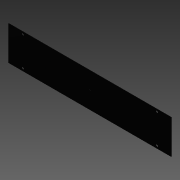
# Autodesk Inventor part: Sheild Flat
Saved by Autodesk Inventor 2014 SP1 (Build 180222100, 222)
## iProperties
Created: 2014-01-13
Part Number: Sheild Flat
Material: Aluminum 6061
Document SubType Name: Sheet Metal
Designer: Rauhul Varma
Mass: 21.0227 g
Surface Area: 199.954 cm^2
Volume: 7.75744 cm^3
Density: 2.71 g/cm^3
Sheet Metal Rule: Default
Appearance: Anodized - Black
Author: Rauhul Varma
Autodesk Inventor part; units mm, degrees
ref_plane "YZ Plane" through (0, 0, 0) normal (1, 0, 0) x (0, 1, 0)
ref_plane "XZ Plane" through (0, 0, 0) normal (0, 1, 0) x (-1, 0, 0)
ref_plane "XY Plane" through (0, 0, 0) normal (0, 0, 1) x (1, 0, 0)
sketch "Sketch1" plane through (0, 0, 0) normal (0, 0, 1) x (1, 0, 0)
  line L0 (0, 0) -> (216.6575, 0)
  line L1 (216.6575, 0) -> (216.6575, 45.2438)
  line L2 (216.6575, 45.2438) -> (0, 45.2437)
  line L3 (0, 45.2437) -> (0, 0)
  dimension "d0" = 216.6575
  dimension "d1" = 45.2437
  measures "d0" distance of L1.end L2.end
  measures "d1" distance of L2.end L0.start
extrude "Plate1" add sketch "Sketch1" along normal blind 0.7937
sketch "Sketch2" plane through (0, 0, 0) normal (0, 0, -1) x (-1, 0, 0)
  line L0 (0, 0) -> (-216.6575, 0) projected
  line L1 (0, 45.2437) -> (0, 0) projected
  line L2 (-216.6575, 45.2438) -> (0, 45.2437) projected
  line L3 (-216.6575, 0) -> (-216.6575, 45.2438) projected
  line L4 (-197.6075, 45.2438) -> (-197.6075, 0) construction
  line L5 (-216.6575, 3.175) -> (0, 3.175) construction
  line L6 (-19.05, 0) -> (-19.05, 45.2437) construction
  line L7 (0, 42.0687) -> (-216.6575, 42.0688) construction
  point P0 (-197.6075, 42.0688)
  point P1 (-197.6075, 3.175)
  point P2 (-19.05, 3.175)
  point P3 (-19.05, 42.0687)
  point P4 (-108.3288, 22.6219)
  dimension "d3" = 3.175
  dimension "d4" = 3.175
  dimension "d5" = 19.05
  dimension "d6" = 19.05
  dimension "d7" = 22.6219
  dimension "d8" = 108.3288
  dimension "d9" = 45.2437
  dimension "d10" = 216.6575
  constraints: 16 point on line, 8 end point, 3 perpendicular, 1 horizontal
  measures "d3" distance between parallel lines of L2 L7
  measures "d4" distance between parallel lines of L0 L5
  measures "d5" distance between parallel lines of L3 L4
  measures "d6" distance between parallel lines of L1 L6
  measures "d7" distance from line of L2 point (-108.329, 22.622)
  measures "d8" distance from line of L1 point (-108.329, 22.622)
  measures "d9" distance of L1.start L0.start
  measures "d10" distance of L2.start L1.start
hole "Hole1" at (197.6075, 42.0688, 0) at (197.6075, 3.175, 0) at (19.05, 3.175, 0) at (19.05, 42.0687, 0) direction (0, 0, 1) diameter 2.9464 end through all clearance for "Flat Head Machine Screw (82)" size "#4" standard "Ansi Unified Screw Threads"
hole "Hole2" at (108.3288, 22.6219, 0) direction (0, 0, 1) diameter 1.5875 end through all
equation "\"d4\" = d3"
equation "\"d6\" = d5"
equation "\"d7\" = 0.5 * d9"
equation "\"d8\" = 0.5 * d10"
equation "\"d16\" = Thickness"
equation "\"d23\" = Thickness"
equation "\"BendRadius\" = Thickness"
equation "\"BendReliefWidth\" = Thickness"
equation "\"BendReliefDepth\" = 0.5 * Thickness"
equation "\"CornerReliefSize\" = 4 * Thickness"
equation "\"MinimumRemnant\" = 2 * Thickness"
equation "\"TransitionRadius\" = BendRadius"
equation "\"JacobiRadiusSize\" = BendRadius"
equation "\"GapSize\" = Thickness"
equation "\"d2\" = BendRadius"
equation "\"Thickness\" = 0.79375"
body "Solid1"
